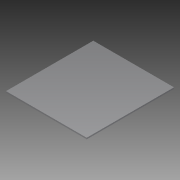
# Autodesk Inventor part: Backboard
Saved by Autodesk Inventor 2013 (Build 170138000, 138)
## iProperties
Created: 2013-01-27
Part Number: Backboard
Material: Polycarbonate, Clear
Document SubType Name: Modeling
Designer: Andrew Toennies
Density: 1.2 g/cm^3
Mass: 149.517 g
Surface Area: 810.042 cm^2
Volume: 124.597 cm^3
Author: Andrew Toennies
Autodesk Inventor part; units mm, degrees
ref_plane "YZ Plane" through (0, 0, 0) normal (1, 0, 0) x (0, 1, 0)
ref_plane "XZ Plane" through (0, 0, 0) normal (0, 1, 0) x (-1, 0, 0)
ref_plane "XY Plane" through (0, 0, 0) normal (0, 0, 1) x (1, 0, 0)
sketch "Sketch1" plane through (0, 0, 0) normal (0, 1, 0) x (-1, 0, 0)
  line L0 (0, 0) -> (0, 206.0011)
  line L1 (0, 0) -> (190.5, 0)
  line L2 (0, 206.0011) -> (190.5, 206.0011)
  line L3 (190.5, 206.0011) -> (190.5, 0)
  dimension "d0" = 206.0011
  dimension "d1" = 190.5
  dimension "d4" = 190.5
  constraints: 8 end point, 1 parallel, 1 perpendicular, 1 vertical
  measures "d0" distance of L0.start L0.end
  measures "d1" distance of L0.start L1.end
  measures "d4" distance of L0.end L2.end
extrude "Extrusion1" add sketch "Sketch1" along normal blind 3.175
body "Solid1"
